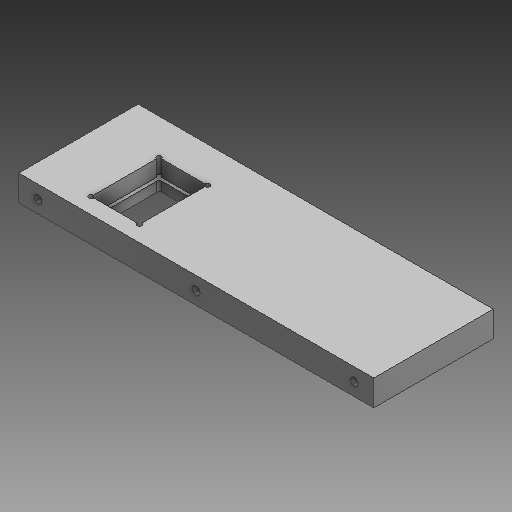
# Autodesk Inventor part: side
Saved by Autodesk Inventor 2019 (Build 230136000, 136)
## iProperties
Created: 2018-05-03
Part Number: side
Material: Aluminum 6061
Document SubType Name: Modeling
Designer: SimonD
Density: 2.7 g/cm^3
Appearance: Aluminum - Polished
Author: SimonD
Autodesk Inventor part; units mm, degrees
ref_plane "YZ Plane" through (0, 0, 0) normal (1, 0, 0) x (0, 1, 0)
ref_plane "XZ Plane" through (0, 0, 0) normal (0, 1, 0) x (-1, 0, 0)
ref_plane "XY Plane" through (0, 0, 0) normal (0, 0, 1) x (1, 0, 0)
sketch "Sketch1" plane through (0, 0, 0) normal (0, 0, 1) x (1, 0, 0)
  line L0 (-55, 4) -> (55, 4)
  line L1 (55, 4) -> (55, -4)
  line L2 (55, -4) -> (-55, -4)
  line L3 (-55, -4) -> (-55, 4)
  line L4 (-55, 4) -> (55, -4) construction
  line L5 (55, 4) -> (-55, -4) construction
  point P0 (0, 0)
  dimension "d0" = 110
  dimension "d1" = 8
  constraints: 12 end point, 2 midpoint, 2 parallel, 1 horizontal, 1 perpendicular
  measures "d0" distance of L1.end L2.end
  measures "d1" distance between parallel lines of L2 L0
extrude "Extrusion1" add sketch "Sketch1" along normal blind 37
sketch "Sketch2" plane through (0, 0, 37) normal (0, 0, 1) x (1, 0, 0)
  line L0 (-55, 4) -> (-55, -4) projected
  line L1 (55, -4) -> (55, 4) projected
  point P0 (0, 0)
  point P1 (-49, 0)
  point P2 (0, 0)
  point P3 (49, 0)
  dimension "d4" = 6
  dimension "d5" = 6
  constraints: 1 coincident
  measures "d4" distance from line of point (-49, 0) L0
  measures "d5" distance from line of L1 point (49, 0)
hole "Hole1" at (-49, 0, 37) at (0, 0, 37) at (49, 0, 37) direction (0, 0, -1) diameter 2.459 depth 8 tip angle 118 thread size "M3x0.5" class "6H" standard "ISO Metric profile"
sketch "Sketch3" plane through (0, 0, 0) normal (0, 0, -1) x (-1, 0, 0)
  circle A0 centre (-49, 0) radius 1.2295 projected
  circle A1 centre (0, 0) radius 1.2295 projected
  circle A2 centre (49, 0) radius 1.2295 projected
  constraints: 3 coincident
hole "Hole2" at (49, 0, 0) at (0, 0, 0) at (-49, 0, 0) direction (0, 0, 1) diameter 2.459 depth 8.8 tip angle 118 thread size "M3x0.5" class "6H" standard "ISO Metric profile"
sketch "Sketch4" plane through (-55, -4, 0) normal (0, -1, 0) x (1, 0, 0)
  line L0 (18.55, 31.1) -> (31.45, 31.1)
  line L1 (31.45, 31.1) -> (31.45, 12)
  line L2 (31.45, 12) -> (18.55, 12)
  line L3 (18.55, 12) -> (18.55, 31.1)
  line L4 (18.55, 31.1) -> (31.45, 12) construction
  line L5 (31.45, 31.1) -> (18.55, 12) construction
  line L6 (110, 0) -> (0, 0) projected
  line L7 (0, 0) -> (0, 37) projected
  line L8 (110, 0) -> (110, 37) projected
  point P0 (55, 0)
  point P1 (25, 21.55)
  dimension "d21" = 12.9
  dimension "d22" = 19.1
  dimension "d23" = 12
  dimension "d29" = 85
  constraints: 12 end point, 2 midpoint, 2 parallel, 1 horizontal, 1 perpendicular
  measures "d21" distance between parallel lines of L1 L3
  measures "d22" distance between parallel lines of L2 L0
  measures "d23" distance between parallel lines of L2 L6
  measures "d29" distance from line of point (25, 21.55) L8
extrude "Extrusion2" cut sketch "Sketch4" against normal blind 10
fillet "Fillet3" radius 0.75 4 edges at (-23.55, 0, 31.1) (-36.45, 0, 31.1) (-36.45, 0, 12) (-23.55, 0, 12)
sketch "Sketch5" plane through (-55, 4, 0) normal (0, 1, 0) x (1, 0, 0)
  line L0 (30.7, -31.1) -> (19.3, -31.1) projected
  line L1 (31.45, -12.75) -> (31.45, -30.35) projected
  line L2 (32.5, -32.05) -> (17.5, -32.05)
  line L3 (17.5, -32.05) -> (17.5, -11.05)
  line L4 (17.5, -11.05) -> (32.5, -11.05)
  line L5 (32.5, -11.05) -> (32.5, -32.05)
  line L6 (32.5, -32.05) -> (17.5, -11.05) construction
  line L7 (17.5, -32.05) -> (32.5, -11.05) construction
  point P0 (55, 0)
  point P1 (25, -21.55)
  dimension "d33" = 9.55
  dimension "d34" = 6.45
  dimension "d35" = 15
  dimension "d36" = 21
  constraints: 12 end point, 2 midpoint, 2 parallel, 1 horizontal, 1 perpendicular
  measures "d33" distance from line of point (25, -21.55) L0
  measures "d34" distance from line of point (25, -21.55) L1
  measures "d35" distance of L3.end L4.end
  measures "d36" distance between parallel lines of L4 L2
extrude "Extrusion3" cut sketch "Sketch5" against normal blind 5
sketch "Sketch6" plane through (-55, 4, 0) normal (0, 1, 0) x (1, 0, 0)
  line L0 (32.5, -32.05) -> (17.5, -32.05) projected
  line L1 (17.5, -32.05) -> (17.5, -11.05) projected
  line L2 (17.5, -11.05) -> (32.5, -11.05) projected
  point P0 (55, 0)
  constraints: 1 coincident
hole "Hole3" at (-22.5, 4, 32.05) at (-37.5, 4, 32.05) at (-37.5, 4, 11.05) at (-22.5, 4, 11.05) direction (0, -1, 0) diameter 1.5 depth 5
body "Solid1"
